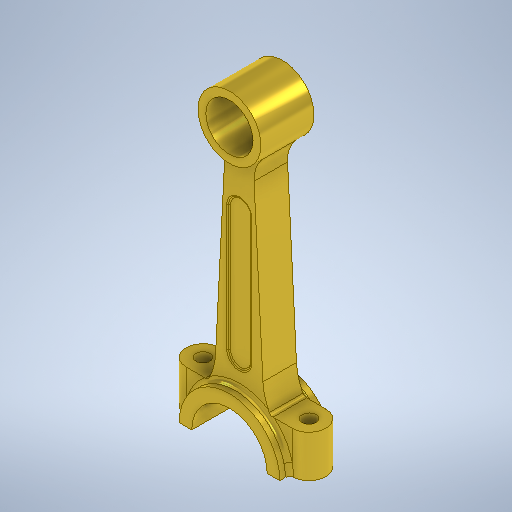
# Autodesk Inventor part: Part 3 Connecting rod
Saved by Autodesk Inventor 2025.2 (Build 292293000, 293)
## iProperties
Created: 2025-03-19
Part Number: Part 3 Connecting rod
Material: Stainless Steel
Document SubType Name: Sheet Metal
Designer: User
Density: 8 g/cm^3
Sheet Metal Rule: Default_mm
Appearance: Metal 2400F Hot
Author: User
Autodesk Inventor part; units mm, degrees
ref_plane "YZ Plane" through (0, 0, 0) normal (1, 0, 0) x (0, 1, 0)
sketch "Sketch1" plane through (0, 0, 0) normal (0, 0, 1) x (1, 0, 0)
  circle A0 centre (0, 94.1694) radius 22.5
  circle A1 centre (0, 94.1694) radius 16.9
  arc A2 (36, -107.0306) -> (-36, -107.0306) centre (0, -107.0306) ccw
  arc A3 (27, -107.0306) -> (-27, -107.0306) centre (0, -107.0306) ccw
  line L0 (-10, 74.0137) -> (-17.8497, -75.7674)
  line L1 (0, -107.0306) -> (0, 94.1694) construction
  line L2 (10, 74.0137) -> (17.8497, -75.7674)
  line L3 (-36, -107.0306) -> (-27, -107.0306)
  line L4 (27, -107.0306) -> (36, -107.0306)
  point P0 (0, 0)
  point P1 (17.8497, -75.7674)
  dimension "d0" = 45
  dimension "d1" = 33.8
  dimension "d2" = 72
  dimension "d3" = 54
  dimension "d4" = 201.2
  dimension "d6" = 3
  dimension "d7" = 6
  constraints: 10 end point, 5 point on circle, 3 centre point, 2 coincident, 2 horizontal, 2 symmetric about line, 1 vertical, 3 other
  measures "d1" diameter of A1
  measures "d2" diameter of A2
  measures "d3" diameter of A3
  measures "d4" distance of A2.centre point (0, 94.169)
  measures "d6" angle of L0 L1
  measures "d7" angle of L0 L2
extrude "Extrusion1" add sketch "Sketch1" along normal mid plane 38 contours A0 | A2 L4 A3 L3
extrude "Extrusion2" add sketch "Sketch1" along normal mid plane 24 contours A0 L2 A2 L0
fillet "Fillet1" radius 40 2 edges at (17.8497, -75.7674, 0) (-17.8497, -75.7674, 0)
fillet "Fillet2" radius 22.5 2 edges at (10, 74.0137, 0) (-10, 74.0137, 0)
sketch "Sketch2" plane through (0, 0, 12) normal (0, 0, 1) x (1, 0, 0)
  circle A0 centre (0, 94.1694) radius 16.9 projected
  arc A1 (27, -107.0306) -> (-27, -107.0306) centre (0, -107.0306) ccw projected
  line L0 (0, 94.1694) -> (0, -107.0306) construction
  line L1 (0, 38.5694) -> (0, -51.4306) construction
  line L2 (-8, 38.5694) -> (-8, -51.4306)
  line L3 (8, -51.4306) -> (8, 38.5694)
  arc A2 (8, 38.5694) -> (-8, 38.5694) centre (0, 38.5694) ccw
  arc A3 (-8, -51.4306) -> (8, -51.4306) centre (0, -51.4306) ccw
  point P0 (0, 0)
  point P1 (0, -6.4306)
  dimension "d14" = 90
  dimension "d15" = 8
  dimension "d16" = 55.6
  constraints: 10 end point, 4 point on circle, 4 tangent, 2 centre point, 2 point on line, 1 midpoint, 1 parallel, 1 vertical
  measures "d14" distance of L3.start L3.end
  measures "d15" radius of A2
  measures "d16" vertical distance of L0.start L3.end
extrude "Extrusion3" cut sketch "Sketch2" against normal blind 1 contours A2 L3 A3 L2
ref_plane "Work Plane1" through (0, 0, 0) normal (0, 0, 1) x (1, 0, 0)
mirror "Mirror1" about plane through (0, 0, 0) normal (0, 0, 1) of "Extrusion3"
fillet "Fillet3" radius 1 16 edges at (8, -6.4306, 12) (0, -59.4306, 12) (-8, -6.4306, 12) (0, 46.5694, 12) (8, -6.4306, 11) (0, -59.4306, 11) (-8, -6.4306, 11) (0, 46.5694, 11) (-8, -6.4306, -12) (0, -59.4306, -12) (8, -6.4306, -12) (0, 46.5694, -12) (8, -6.4306, -11) (0, -59.4306, -11) (-8, -6.4306, -11) (0, 46.5694, -11)
ref_plane "Work Plane2" through (27, -77.0306, 19) normal (0, -1, 0) x (1, 0, 0)
sketch "Sketch3" plane through (27, -77.0306, 19) normal (0, -1, 0) x (1, 0, 0)
  line L0 (0, -38) -> (-54, -38) projected
  line L1 (9, 0) -> (9, -38) projected
  line L2 (11, -19) -> (-65, -19) construction
  line L3 (11, -7) -> (-65, -7)
  line L4 (-65, -31) -> (11, -31)
  arc A0 (11, -31) -> (11, -7) centre (11, -19) ccw
  arc A1 (-65, -7) -> (-65, -31) centre (-65, -19) ccw
  point P0 (-27, -19)
  point P1 (-27, -19)
  point P2 (23, -19)
  point P3 (9, -19)
  point P4 (-27, -38)
  dimension "d21" = 76
  dimension "d22" = 12
  constraints: 8 end point, 5 point on circle, 4 tangent, 3 midpoint, 2 centre point, 1 horizontal, 1 horizontal alignment, 1 parallel, 1 vertical alignment
  measures "d21" distance of L4.start L4.end
  measures "d22" radius of A1
extrude "Extrusion4" add sketch "Sketch3" along normal up to surface (30 mm away)
sketch "Sketch4" plane through (0, -107.0306, -12) normal (0, 0, -1) x (-1, 0, 0)
  arc A0 (27, 0) -> (-27, 0) centre (0, 0) ccw projected
  line L0 (-27, 0) -> (27, 0) projected
  point P0 (0, 107.0306)
extrude "Extrusion5" cut sketch "Sketch4" against normal through all
fillet "Fillet4" radius 3 4 edges at (0, -71.0306, -12) (-22.4835, -77.0306, 0) (0, -71.0306, 12) (22.4835, -77.0306, 0)
sketch "Sketch5" plane through (-36, -107.0306, 19) normal (0, -1, 0) x (1, 0, 0)
  arc A0 (-2.8, -7.0267) -> (-2.8, -30.9733) centre (-2, -19) ccw projected
  point P0 (36, -19)
  constraints: 1 coincident
hole "Hole1" at (-38, -107.0306, 0) direction (0, 1, 0) diameter 10 end through all
sketch "Sketch6" plane through (27, -107.0306, -19) normal (0, -1, 0) x (1, 0, 0)
  arc A0 (11.8, 7.0267) -> (11.8, 30.9733) centre (11, 19) ccw projected
  point P0 (-27, 19)
  constraints: 1 coincident
hole "Hole2" at (38, -107.0306, 0) direction (0, 1, 0) diameter 10 end through all
equation "\"d33\" = Thickness"
equation "\"BendRadius\" = Thickness"
equation "\"BendReliefWidth\" = Thickness"
equation "\"BendReliefDepth\" = 0.5 * Thickness"
equation "\"CornerReliefSize\" = 4 * Thickness"
equation "\"MinimumRemnant\" = 2 * Thickness"
equation "\"TransitionRadius\" = BendRadius"
equation "\"JacobiRadiusSize\" = BendRadius"
equation "\"GapSize\" = Thickness"
equation "\"Thickness\" = 0.5"
body "Solid1"
